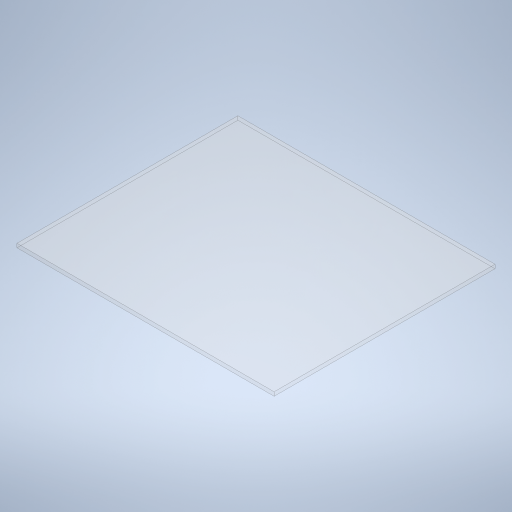
# Autodesk Inventor part: 下板
Saved by Autodesk Inventor 2023 (Build 270158000, 158)
## iProperties
Created: 2022-05-13
Part Number: 下板
Material: ポリカーボネート、クリア
Document SubType Name: Modeling
Designer: muzho
Density: 1.2 g/cm^3
Appearance: ポリカーボネート - クリア
Author: muzho
Autodesk Inventor part; units mm, degrees
ref_plane "YZ Plane" through (0, 0, 0) normal (1, 0, 0) x (0, 1, 0)
ref_plane "XZ Plane" through (0, 0, 0) normal (0, 1, 0) x (-1, 0, 0)
ref_plane "XY Plane" through (0, 0, 0) normal (0, 0, 1) x (1, 0, 0)
sketch "スケッチ1" plane through (0, 0, 0) normal (0, 1, 0) x (-1, 0, 0)
  line L0 (78.62, 78.1674) -> (-119.28, 78.1674)
  line L1 (78.62, 78.1674) -> (78.62, -91.8326)
  line L2 (78.62, -91.8326) -> (-119.28, -91.8326)
  line L3 (-119.28, -91.8326) -> (-119.28, 78.1674)
  point P0 (0, 0)
  dimension "d0" = 197.9
  dimension "d1" = 170
  constraints: 8 end point, 2 horizontal, 1 perpendicular, 1 vertical
  measures "d0" distance of L0.start L0.end
  measures "d1" distance of L0.start L1.end
extrude "押し出し1" add sketch "スケッチ1" along normal blind 3
